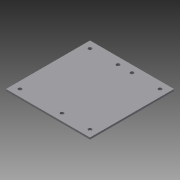
# Autodesk Inventor part: pickup arm plate
Saved by Autodesk Inventor 2015 (Build 190159000, 159)
## iProperties
Created: 2015-01-27
Part Number: pickup arm plate
Material: Generic
Document SubType Name: Modeling
Designer: Admin
Density: 1 g/cm^3
Appearance: Default
Author: Admin
Autodesk Inventor part; units mm, degrees
ref_plane "YZ Plane" through (0, 0, 0) normal (1, 0, 0) x (0, 1, 0)
ref_plane "XZ Plane" through (0, 0, 0) normal (0, 1, 0) x (-1, 0, 0)
ref_plane "XY Plane" through (0, 0, 0) normal (0, 0, 1) x (1, 0, 0)
sketch "Sketch1" plane through (0, 0, 0) normal (0, 1, 0) x (-1, 0, 0)
  line L0 (0, 0) -> (152.4, 0)
  line L1 (152.4, 0) -> (152.4, -152.4)
  line L2 (152.4, -152.4) -> (0, -152.4)
  line L3 (0, -152.4) -> (0, 0)
  dimension "d0" = 152.4
  dimension "d1" = 152.4
  constraints: 8 end point, 2 parallel, 1 horizontal, 1 perpendicular
  measures "d0" distance of L1.end L2.end
  measures "d1" distance of L0.end L1.end
extrude "Extrusion1" add sketch "Sketch1" along normal blind 3.175
sketch "Sketch2" plane through (0, 3.175, 0) normal (0, 1, 0) x (1, 0, 0)
  line L0 (-152.4, 0) -> (0, 0) projected
  line L1 (0, 0) -> (0, 152.4) projected
  line L2 (0, 152.4) -> (-152.4, 152.4) projected
  line L3 (-152.4, 152.4) -> (-152.4, 0) projected
  point P0 (-139.7, 12.7)
  point P1 (-63.5, 12.7)
  point P2 (-12.7, 12.7)
  point P3 (-12.7, 139.7)
  point P4 (-63.5, 139.7)
  point P5 (-139.7, 139.7)
  dimension "d4" = 12.7
  dimension "d5" = 12.7
  dimension "d6" = 12.7
  dimension "d7" = 12.7
  dimension "d8" = 12.7
  dimension "d9" = 12.7
  dimension "d10" = 12.7
  dimension "d11" = 63.5
  dimension "d12" = 12.7
  dimension "d13" = 12.7
  dimension "d14" = 12.7
  dimension "d15" = 63.5
  measures "d4" distance from line of L0 point (-139.7, 12.7)
  measures "d5" distance from line of L3 point (-139.7, 12.7)
  measures "d6" distance from line of L3 point (-139.7, 139.7)
  measures "d7" distance from line of L2 point (-139.7, 139.7)
  measures "d8" distance from line of L1 point (-12.7, 12.7)
  measures "d9" distance from line of L0 point (-12.7, 12.7)
  measures "d10" distance from line of L0 point (-63.5, 12.7)
  measures "d11" distance from line of L1 point (-63.5, 12.7)
  measures "d12" distance from line of L1 point (-12.7, 139.7)
  measures "d13" distance from line of L2 point (-12.7, 139.7)
  measures "d14" distance from line of L2 point (-63.5, 139.7)
  measures "d15" distance from line of L1 point (-63.5, 139.7)
hole "Hole1" at (-139.7, 3.175, -12.7) at (-63.5, 3.175, -12.7) at (-12.7, 3.175, -12.7) at (-12.7, 3.175, -139.7) at (-63.5, 3.175, -139.7) at (-139.7, 3.175, -139.7) direction (0, -1, 0) diameter 6.35 end through all
sketch "Sketch3" plane through (0, 3.175, 0) normal (0, 1, 0) x (1, 0, 0)
  circle A0 centre (-139.7, 139.7) radius 3.175 projected
  line L0 (0, 152.4) -> (-152.4, 152.4) projected
  point P0 (-88.9, 139.7)
  dimension "d23" = 12.7
  dimension "d24" = 50.8
  measures "d23" distance from line of L0 point (-88.9, 139.7)
  measures "d24" distance of point (-88.9, 139.7) A0.centre
hole "Hole2" at (-88.9, 3.175, -139.7) direction (0, -1, 0) diameter 6.35 end through all
body "Solid1"
